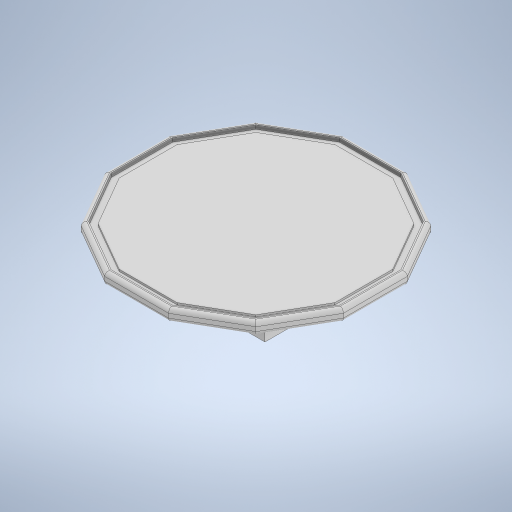
# Autodesk Inventor part: OV-PAM_n_12_bottom
Saved by Autodesk Inventor 2024 (Build 280153000, 153)
## iProperties
Created: 2023-08-31
Part Number: OV-PAM_n_12_bottom
Material: 일반
Document SubType Name: Modeling
Designer: jsw
Density: 1 g/cm^3
Appearance: 기본값
Author: jsw
Autodesk Inventor part; units mm, degrees
ref_plane "YZ Plane" through (0, 0, 0) normal (1, 0, 0) x (0, 1, 0)
ref_plane "XZ Plane" through (0, 0, 0) normal (0, 1, 0) x (-1, 0, 0)
ref_plane "XY Plane" through (0, 0, 0) normal (0, 0, 1) x (1, 0, 0)
sketch "스케치1" plane through (0, 0, 0) normal (0, 1, 0) x (-1, 0, 0)
  line L0 (24.9446, -24.9446) -> (9.1304, -34.075)
  line L1 (9.1304, -34.075) -> (-9.1304, -34.075)
  line L2 (-9.1304, -34.075) -> (-24.9446, -24.9446)
  line L3 (-24.9446, -24.9446) -> (-34.075, -9.1304)
  line L4 (-34.075, -9.1304) -> (-34.075, 9.1304)
  line L5 (-34.075, 9.1304) -> (-24.9446, 24.9446)
  line L6 (-24.9446, 24.9446) -> (-9.1304, 34.075)
  line L7 (-9.1304, 34.075) -> (9.1304, 34.075)
  line L8 (9.1304, 34.075) -> (24.9446, 24.9446)
  line L9 (24.9446, 24.9446) -> (34.075, 9.1304)
  line L10 (34.075, 9.1304) -> (34.075, -9.1304)
  line L11 (34.075, -9.1304) -> (24.9446, -24.9446)
  line L12 (9.9878, -37.275) -> (-9.9878, -37.275)
  line L13 (-9.9878, -37.275) -> (-27.2872, -27.2872)
  line L14 (-27.2872, -27.2872) -> (-37.275, -9.9878)
  line L15 (-37.275, -9.9878) -> (-37.275, 9.9878)
  line L16 (-37.275, 9.9878) -> (-27.2872, 27.2872)
  line L17 (-27.2872, 27.2872) -> (-9.9878, 37.275)
  line L18 (-9.9878, 37.275) -> (9.9878, 37.275)
  line L19 (9.9878, 37.275) -> (27.2872, 27.2872)
  line L20 (27.2872, 27.2872) -> (37.275, 9.9878)
  line L21 (37.275, 9.9878) -> (37.275, -9.9878)
  line L22 (37.275, -9.9878) -> (27.2872, -27.2872)
  line L23 (27.2872, -27.2872) -> (9.9878, -37.275)
  point P0 (0, 0)
  point P1 (0, 0)
  point P2 (0, 0)
  dimension "d0" = 70.554
  dimension "d1" = 3.2
  constraints: 48 end point, 2 coincident, 2 horizontal, 50 other
  measures "d0" distance of L3.end L9.end
  measures "d1" distance between parallel lines of L10 L21
extrude "돌출1" add sketch "스케치1" along normal blind 3.7 contours L0 L1 L2 L3 L4 L5 L6 L7 L8 L9 L10 L11 | L12 L13 L14 L15 L16 L17 L18 L19 L20 L21 L22 L23
sketch "스케치2" plane through (0, 3.7, 0) normal (0, 1, 0) x (1, 0, 0)
  line L0 (-9.5591, 35.675) -> (9.5591, 35.675)
  line L1 (9.5591, 35.675) -> (26.1159, 26.1159)
  line L2 (26.1159, 26.1159) -> (35.675, 9.5591)
  line L3 (35.675, 9.5591) -> (35.675, -9.5591)
  line L4 (35.675, -9.5591) -> (26.1159, -26.1159)
  line L5 (26.1159, -26.1159) -> (9.5591, -35.675)
  line L6 (9.5591, -35.675) -> (-9.5591, -35.675)
  line L7 (-9.5591, -35.675) -> (-26.1159, -26.1159)
  line L8 (-26.1159, -26.1159) -> (-35.675, -9.5591)
  line L9 (-35.675, -9.5591) -> (-35.675, 9.5591)
  line L10 (-35.675, 9.5591) -> (-26.1159, 26.1159)
  line L11 (-26.1159, 26.1159) -> (-9.5591, 35.675)
  line L12 (9.9878, 37.275) -> (-9.9878, 37.275) projected
  point P0 (0, 0)
  point P1 (0, 0)
  point P2 (0, 35.675)
  dimension "d4" = 1.6
  constraints: 24 end point, 1 coincident, 1 horizontal, 1 midpoint, 25 other
  measures "d4" distance from line of L12 point (0, 35.675)
extrude "돌출2" cut sketch "스케치2" against normal blind 1.2
sketch "스케치3" plane through (0, 2.5, 0) normal (0, 1, 0) x (1, 0, 0)
  line L0 (-9.0232, 33.675) -> (9.0232, 33.675)
  line L1 (9.0232, 33.675) -> (24.6518, 24.6518)
  line L2 (24.6518, 24.6518) -> (33.675, 9.0232)
  line L3 (33.675, 9.0232) -> (33.675, -9.0232)
  line L4 (33.675, -9.0232) -> (24.6518, -24.6518)
  line L5 (24.6518, -24.6518) -> (9.0232, -33.675)
  line L6 (9.0232, -33.675) -> (-9.0232, -33.675)
  line L7 (-9.0232, -33.675) -> (-24.6518, -24.6518)
  line L8 (-24.6518, -24.6518) -> (-33.675, -9.0232)
  line L9 (-33.675, -9.0232) -> (-33.675, 9.0232)
  line L10 (-33.675, 9.0232) -> (-24.6518, 24.6518)
  line L11 (-24.6518, 24.6518) -> (-9.0232, 33.675)
  line L12 (-9.5591, 35.675) -> (9.5591, 35.675) projected
  point P0 (0, 0)
  point P1 (0, 0)
  dimension "d7" = 2
  constraints: 24 end point, 1 coincident, 1 horizontal, 25 other
  measures "d7" distance between parallel lines of L12 L0
extrude "돌출3" add sketch "스케치3" along normal blind 0.6
fillet "모깎기1" radius 1.2 24 edges at (-18.6375, 3.7, 32.2811) (-32.2811, 3.7, 18.6375) (-37.275, 3.7, 0) (0, 3.7, 37.275) (18.6375, 3.7, 32.2811) (32.2811, 3.7, 18.6375) (37.275, 3.7, 0) (32.2811, 3.7, -18.6375) (18.6375, 3.7, -32.2811) (0, 3.7, -37.275) (-18.6375, 3.7, -32.2811) (-32.2811, 3.7, -18.6375) (-37.275, 0, 0) (-32.2811, 0, 18.6375) (-18.6375, 0, 32.2811) (0, 0, 37.275) (18.6375, 0, 32.2811) (32.2811, 0, 18.6375) (37.275, 0, 0) (32.2811, 0, -18.6375) (18.6375, 0, -32.2811) (0, 0, -37.275) (-18.6375, 0, -32.2811) (-32.2811, 0, -18.6375)
sketch "스케치10" plane through (0, 0, 0) normal (0, -1, 0) x (1, 0, 0)
  line L0 (10.3, 12.5) -> (15.3, 12.5)
  line L1 (15.3, 12.5) -> (15.3, -12.5)
  line L2 (15.3, -12.5) -> (10.3, -12.5)
  line L3 (10.3, -12.5) -> (10.3, 12.5)
  line L4 (10.3, 12.5) -> (15.3, -12.5) construction
  line L5 (15.3, 12.5) -> (10.3, -12.5) construction
  line L6 (0, 0) -> (0, -4.638)
  line L7 (-10.3, 12.5) -> (-15.3, 12.5)
  line L8 (-15.3, 12.5) -> (-15.3, -12.5)
  line L9 (-15.3, -12.5) -> (-10.3, -12.5)
  line L10 (-10.3, -12.5) -> (-10.3, 12.5)
  line L11 (-10.3, 12.5) -> (-15.3, -12.5) construction
  line L12 (-15.3, 12.5) -> (-10.3, -12.5) construction
  point P0 (12.8, 0)
  point P1 (-12.8, 0)
  dimension "d50" = 5
  dimension "d51" = 25
  dimension "d52" = 10.3
  constraints: 26 end point, 5 symmetric about line, 2 midpoint, 2 parallel, 1 horizontal, 1 horizontal alignment, 1 perpendicular, 1 vertical
  measures "d50" distance of L1.end L2.end
  measures "d51" distance of L0.end L1.end
  measures "d52" distance from line of L6.start L3
extrude "돌출7" add sketch "스케치10" along normal blind 15
sketch "스케치11" plane through (15.3, 0, 12.5) normal (1, 0, 0) x (0, 0, -1)
  circle A0 centre (7.5, -7.5) radius 1.25
  line L0 (2.8337, 0) -> (22.1663, 0) projected
  line L1 (12.5, 0) -> (12.5, -3.2899)
  circle A1 centre (17.5, -7.5) radius 1.25
  point P0 (12.5, 0)
  dimension "d55" = 2.5
  dimension "d56" = 7.5
  dimension "d57" = 5
  constraints: 2 centre point, 2 end point, 1 midpoint, 1 symmetric about line, 1 vertical, 1 other
  measures "d55" diameter of A0
  measures "d56" distance from line of L0 A0.centre
  measures "d57" horizontal distance of A0.centre L1.start
extrude "돌출8" cut sketch "스케치11" against normal up to surface (30.6 mm away)
equation "\"d38\" = 55deg"
